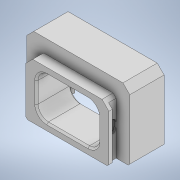
# Autodesk Inventor part: Nikon-D3400-DK-25-Extension - Inventor
Saved by Autodesk Inventor 2020.2 (Build 242310000, 310)
## iProperties
Created: 2020-02-29
Part Number: Nikon-D3400-DK-25-Extension - Inventor
Material: Generic
Document SubType Name: Modeling
Designer: roota
Density: 1 g/cm^3
Appearance: Default
Author: roota
Autodesk Inventor part; units mm, degrees
ref_plane "YZ Plane" through (0, 0, 0) normal (1, 0, 0) x (0, 1, 0)
ref_plane "XZ Plane" through (0, 0, 0) normal (0, 1, 0) x (-1, 0, 0)
ref_plane "XY Plane" through (0, 0, 0) normal (0, 0, 1) x (1, 0, 0)
sketch "Sketch1" plane through (0, 0, 0) normal (0, 0, 1) x (1, 0, 0)
  line L0 (-15, -10) -> (15, -10)
  line L1 (15, -10) -> (15, 10)
  line L2 (15, 10) -> (-15, 10)
  line L3 (-15, 10) -> (-15, -10)
  line L4 (-15, -10) -> (15, 10) construction
  line L5 (15, -10) -> (-15, 10) construction
  line L6 (-9, -8) -> (9, -8)
  line L7 (9, -8) -> (9, 4)
  line L8 (9, 4) -> (-9, 4)
  line L9 (-9, 4) -> (-9, -8)
  point P0 (0, 0)
  point P1 (0, 0)
  point P2 (0, -8)
  dimension "d0" = 30
  dimension "d1" = 20
  dimension "d2" = 18
  dimension "d3" = 12
  dimension "d13" = 2
  constraints: 20 end point, 4 midpoint, 4 parallel, 2 horizontal, 2 perpendicular, 1 vertical alignment
  measures "d0" distance of L2.end L1.end
  measures "d1" distance of L1.end L0.end
  measures "d2" distance of L8.end L7.end
  measures "d3" distance of L7.end L6.end
  measures "d13" distance between parallel lines of L0 L6
extrude "Extrusion1" add sketch "Sketch1" along normal blind 7
sketch "Sketch2" plane through (0, 0, 7) normal (0, 0, 1) x (1, 0, 0)
  line L0 (-11, -10) -> (11, -10)
  line L1 (11, -10) -> (11, 6)
  line L2 (11, 6) -> (-11, 6)
  line L3 (-11, 6) -> (-11, -10)
  line L4 (-11, -10) -> (11, 6) construction
  line L5 (11, -10) -> (-11, 6) construction
  line L6 (15, -10) -> (15, 10) projected
  line L7 (-15, -10) -> (15, -10) projected
  line L8 (-15, 10) -> (-15, -10) projected
  line L9 (15, 10) -> (-15, 10) projected
  line L10 (-9, 4) -> (9, 4) projected
  line L11 (-9, -8) -> (-9, 4) projected
  line L12 (9, -8) -> (-9, -8) projected
  line L13 (9, 4) -> (9, -8) projected
  point P0 (0, -2)
  point P1 (0, 0)
  point P2 (0, -2)
  dimension "d6" = 22
  dimension "d7" = 16
  constraints: 12 end point, 3 midpoint, 2 parallel, 1 horizontal, 1 perpendicular, 1 point on line, 1 vertical alignment
  measures "d6" distance of L2.end L1.end
  measures "d7" distance of L1.end L0.end
extrude "Extrusion2" add sketch "Sketch2" along normal blind 2.2 contours L3 L2 L1 L0
sketch "Sketch3" plane through (0, 0, 9.2) normal (0, 0, 1) x (1, 0, 0)
  line L0 (-12.1, -10) -> (12.1, -10)
  line L1 (12.1, -10) -> (12.1, 6)
  line L2 (12.1, 6) -> (-12.1, 6)
  line L3 (-12.1, 6) -> (-12.1, -10)
  line L4 (-12.1, -10) -> (12.1, 6) construction
  line L5 (12.1, -10) -> (-12.1, 6) construction
  line L6 (-9, -8) -> (-9, 4) projected
  line L7 (-9, 4) -> (9, 4) projected
  line L8 (9, -8) -> (-9, -8) projected
  line L9 (9, 4) -> (9, -8) projected
  line L10 (-11, -10) -> (11, -10) projected
  point P0 (0, -2)
  point P1 (11, 6)
  point P2 (0, -10)
  dimension "d10" = 24.2
  constraints: 12 end point, 4 midpoint, 2 parallel, 1 horizontal, 1 perpendicular, 1 point on line
  measures "d10" distance of L2.end L1.end
extrude "Extrusion3" add sketch "Sketch3" along normal blind 1
sketch "Sketch4" plane through (11, -10, 7) normal (1, 0, 0) x (0, 0, -1)
  line L0 (0, 16) -> (0, 0) construction
  line L1 (0, 16) -> (-2.2, 16) construction
  line L2 (-2.2, 0) -> (-2.2, 16) construction
  line L3 (0, 0) -> (-2.2, 0) construction
  line L4 (-2.2, 16) -> (-2.2, 0) construction
  line L5 (0, 20) -> (0, 0) construction
  line L6 (0, 9.2) -> (0, 7.7)
  line L7 (-2.2, 7.7) -> (-2.2, 9.2)
  arc A0 (-2.2, 7.7) -> (0, 7.7) centre (-1.1, 7.7) ccw
  arc A1 (0, 9.2) -> (-2.2, 9.2) centre (-1.1, 9.2) ccw
  point P0 (7, 10)
  dimension "d19" = 6.8
  dimension "d20" = 1.5
  constraints: 4 end point, 4 point on circle, 4 point on line, 4 tangent, 2 centre point, 1 parallel
  measures "d19" distance from line of A1.centre L1
  measures "d20" distance of A0.centre A1.centre
extrude "Extrusion4" cut sketch "Sketch4" against normal blind 0.6
sketch "Sketch5" plane through (0, 0, 0) normal (0, 0, -1) x (-1, 0, 0)
  line L0 (-12.5, -10) -> (12.5, -10)
  line L1 (12.5, -10) -> (12.5, 6)
  line L2 (12.5, 6) -> (-12.5, 6)
  line L3 (-12.5, 6) -> (-12.5, -10)
  line L4 (-12.5, -10) -> (12.5, 6) construction
  line L5 (12.5, -10) -> (-12.5, 6) construction
  line L6 (15, -10) -> (-15, -10) projected
  line L7 (15, 10) -> (15, -10) projected
  line L8 (-15, 10) -> (15, 10) projected
  line L9 (-15, -10) -> (-15, 10) projected
  line L10 (9, -8) -> (9, 4) projected
  line L11 (-9, -8) -> (9, -8) projected
  line L12 (-9, 4) -> (-9, -8) projected
  line L13 (9, 4) -> (-9, 4) projected
  line L14 (15, -10) -> (-15, -10) projected
  point P0 (0, 0)
  point P1 (0, -2)
  point P2 (0, -2)
  dimension "d21" = 25
  dimension "d22" = 16
  constraints: 12 end point, 3 midpoint, 2 parallel, 1 horizontal, 1 perpendicular, 1 point on line, 1 vertical alignment
  measures "d21" distance of L2.end L1.end
  measures "d22" distance of L1.end L0.end
extrude "Extrusion5" add sketch "Sketch5" along normal blind 3 contours L6 L9 L8 L7 L1 L2 L3
sketch "Sketch6" plane through (0, 0, -3) normal (0, 0, -1) x (-1, 0, 0)
  line L0 (-12.5, 6) -> (-12.5, -10) projected
  line L1 (12.1, -10) -> (-12.1, -10) construction
  line L2 (-12.5, 6) -> (-11, 6)
  line L3 (-11, 6) -> (-11, -10)
  line L4 (-11, -10) -> (-12.5, -10)
  line L5 (-12.5, -10) -> (-12.5, 6)
  line L6 (12.5, 6) -> (-12.5, 6) projected
  line L7 (12.5, 6) -> (11, 6)
  line L8 (11, 6) -> (11, -10)
  line L9 (11, -10) -> (12.5, -10)
  line L10 (12.5, -10) -> (12.5, 6)
  line L11 (-11, -0.5) -> (-10.8, -0.7)
  line L12 (-10.8, -0.7) -> (-10.8, -2.3)
  line L13 (-9, 4) -> (-9, -8) construction
  line L14 (-10.8, -2.3) -> (-11, -2.5)
  line L15 (12.5, 6) -> (12.5, -10) projected
  line L16 (12.5, 1) -> (10.8, -0.7)
  line L17 (10.8, -0.7) -> (10.8, -2.3)
  line L18 (11, -10) -> (11, 6) projected
  line L19 (10.8, -2.3) -> (12.5, -4)
  point P0 (0, 0)
  point P1 (11, 6)
  point P2 (11, -0.5)
  point P3 (11, -2.5)
  dimension "d26" = 22
  dimension "d27" = 11
  dimension "d28" = 21.6
  dimension "d29" = 10.8
  dimension "d30" = 45
  dimension "d31" = 45
  dimension "d32" = 45
  dimension "d33" = 45
  dimension "d34" = 7.5
  dimension "d35" = 2
  constraints: 28 end point, 7 parallel, 6 point on line, 2 horizontal, 2 perpendicular, 1 horizontal alignment
  measures "d26" distance between parallel lines of L8 L3
  measures "d27" distance from line of point (0, 0) L3
  measures "d28" distance between parallel lines of L17 L12
  measures "d29" distance from line of point (0, 0) L12
  measures "d30" angle of L3 L11
  measures "d31" angle of L17 L16
  measures "d32" angle of L17 L19
  measures "d33" angle of L12 L14
  measures "d34" distance from line of L4 L14.end
  measures "d35" distance of L14.end L11.start
extrude "Extrusion6" add sketch "Sketch6" against normal blind 1.4
fillet "Fillet3" radius 2 2 edges at (-11, 6, -2.3) (11, 6, -2.3)
fillet "Fillet1" radius 3 6 edges at (-12.5, 6, -0.8) (12.5, 6, -0.8) (-9, 4, 5.1) (9, 4, 5.1) (9, -8, 5.1) (-9, -8, 5.1)
mirror "Mirror1" about plane through (0, 0, 0) normal (1, 0, 0) of "Extrusion4"
chamfer "Chamfer1" distance 2 angle 45 4 edges at (12.1, 6, 9.7) (-12.1, 6, 9.7) (15, 10, 2) (-15, 10, 2)
chamfer "Chamfer2" distance 0.5 angle 45 24 edges at (15, -10, 2) (-15, -10, 2) (-12.1, -10, 9.7) (12.1, -10, 9.7) (11, -10, -2.3) (-11, -10, -2.3) (-12.5, -10, -0.8) (12.5, -10, -0.8) (0, -8, 0) (-8.1213, -7.1213, 0) (-9, -2, 0) (-8.1213, 3.1213, 0) (0, 4, 0) (8.1213, 3.1213, 0) (9, -2, 0) (8.1213, -7.1213, 0) (-8.1213, -7.1213, 10.2) (0, -8, 10.2) (8.1213, -7.1213, 10.2) (9, -2, 10.2) (8.1213, 3.1213, 10.2) (0, 4, 10.2) (-8.1213, 3.1213, 10.2) (-9, -2, 10.2)
sketch "Sketch8" plane through (0, 0, -3) normal (0, 0, -1) x (-1, 0, 0)
  line L0 (-9, 6) -> (9, 6) construction
  line L1 (-11, -0.5) -> (-11, 4) construction
  line L2 (11, 4) -> (11, -0.5) construction
  line L3 (-11, 6) -> (11, 6)
  line L4 (11, 6) -> (11, -0.5)
  line L5 (11, -0.5) -> (-11, -0.5)
  line L6 (-11, -0.5) -> (-11, 6)
  point P0 (0, 0)
  point P1 (-10.1, 6)
  constraints: 8 end point, 2 parallel, 2 point on line, 1 horizontal, 1 perpendicular
extrude "Extrusion7" cut sketch "Sketch8" against normal up to surface (1.4 mm away)
equation "\"d27\" = 0.5 * d26"
equation "\"d29\" = 0.5 * d28"
body "Solid1"
